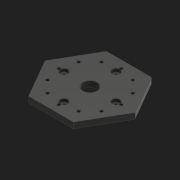
# Autodesk Inventor part: AC04
Saved by Autodesk Inventor 2017 (Build 210142000, 142)
## iProperties
Created: 2019-08-28
Part Number: AC04
Material: ABS Plastic
Document SubType Name: Modeling
Designer: Dell
Density: 1.06 g/cm^3
Appearance: Smooth - Black
Author: Dell
Autodesk Inventor part; units mm, degrees
ref_plane "YZ Plane" through (0, 0, 0) normal (1, 0, 0) x (0, 1, 0)
ref_plane "XZ Plane" through (0, 0, 0) normal (0, 1, 0) x (-1, 0, 0)
ref_plane "XY Plane" through (0, 0, 0) normal (0, 0, 1) x (1, 0, 0)
sketch "Sketch1" plane through (0, 0, 0) normal (0, 0, 1) x (1, 0, 0)
  line L0 (77.9423, 0) -> (38.9711, -67.5)
  line L1 (38.9711, -67.5) -> (-38.9711, -67.5)
  line L2 (-38.9711, -67.5) -> (-77.9423, 0)
  line L3 (-77.9423, 0) -> (-38.9711, 67.5)
  line L4 (-38.9711, 67.5) -> (38.9711, 67.5)
  line L5 (38.9711, 67.5) -> (77.9423, 0)
  circle A0 centre (0, 0) radius 12.5
  circle A1 centre (54, 0) radius 2.5
  circle A2 centre (46.7654, 27) radius 2.5
  circle A3 centre (27, 46.7654) radius 2.5
  circle A4 centre (0, 54) radius 2.5
  circle A5 centre (-27, 46.7654) radius 2.5
  circle A6 centre (-46.7654, 27) radius 2.5
  circle A7 centre (-54, 0) radius 2.5
  circle A8 centre (-46.7654, -27) radius 2.5
  circle A9 centre (-27, -46.7654) radius 2.5
  circle A10 centre (0, -54) radius 2.5
  circle A11 centre (27, -46.7654) radius 2.5
  circle A12 centre (46.7654, -27) radius 2.5
  dimension "d0" = 135
  dimension "d1" = 25
  dimension "d2" = 54
  dimension "d3" = 5
  dimension "d6" = 360
  constraints: 13 centre point, 12 end point, 2 coincident, 2 horizontal alignment, 38 other
  measures "d0" distance between parallel lines of L1 L4
  measures "d1" diameter of A0
  measures "d2" distance of A1.centre point (0, 0)
  measures "d3" diameter of A1
extrude "Extrusion1" add sketch "Sketch1" along normal blind 10
sketch "Sketch2" plane through (0, 0, 10) normal (0, 0, 1) x (1, 0, 0)
  circle A0 centre (0, 45) radius 2.5
  circle A1 centre (-45, 0) radius 2.5
  circle A2 centre (0, -45) radius 2.5
  circle A3 centre (45, 0) radius 2.5
  point P0 (0, 0)
  dimension "d10" = 5
  dimension "d11" = 45
  dimension "d14" = 360
  constraints: 4 centre point, 1 vertical alignment, 9 other
  measures "d10" diameter of A0
  measures "d11" distance of point (0, 0) A0.centre
extrude "Extrusion2" cut sketch "Sketch2" against normal through all
sketch "Sketch4" plane through (0, 0, 10) normal (0, 0, 1) x (1, 0, 0)
  circle A0 centre (0, 45) radius 2.5 projected
  circle A1 centre (0, 45) radius 6.5
  circle A2 centre (-45, 0) radius 6.5
  circle A3 centre (0, -45) radius 6.5
  circle A4 centre (45, 0) radius 6.5
  point P0 (0, 0)
  dimension "d22" = 13
  dimension "d28" = 360
  constraints: 4 centre point, 1 coincident, 9 other
  measures "d22" diameter of A1
extrude "Extrusion4" cut sketch "Sketch4" against normal blind 5
body "Solid1"
